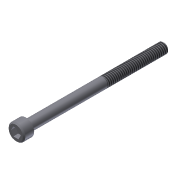
# Autodesk Inventor part: 10-32 x1000
Saved by Autodesk Inventor 2013 (Build 170138000, 138)
## iProperties
Created: 2011-07-11
Part Number: 10-32 x1000
Document SubType Name: Modeling
Designer: Dan Niemitalo
Density: 7.85 g/cm^3
Material: Steel
Mass: 5.59341 g
Surface Area: 6.83094 cm^2
Volume: 0.712536 cm^3
Author: Dan Niemitalo
Autodesk Inventor part; units mm, degrees
ref_plane "YZ Plane" through (0, 0, 0) normal (1, 0, 0) x (0, 1, 0)
ref_plane "XZ Plane" through (0, 0, 0) normal (0, 1, 0) x (-1, 0, 0)
ref_plane "XY Plane" through (0, 0, 0) normal (0, 0, 1) x (1, 0, 0)
sketch "Sketch1" plane through (0, 0, 0) normal (0, 0, 1) x (1, 0, 0)
  circle A0 centre (0, 0) radius 3.429
  dimension "d0" = 6.858
  constraints: 1 centre point, 1 coincident
  measures "d0" diameter of A0
extrude "Extrusion1" add sketch "Sketch1" along normal blind 4.1656
sketch "Sketch2" plane through (0, 0, 0) normal (0, 0, -1) x (-1, 0, 0)
  circle A0 centre (0, 0) radius 3.429 projected
  circle A1 centre (0, 0) radius 2.0828
  dimension "d3" = 4.1656
  constraints: 1 centre point, 1 coincident
  measures "d3" diameter of A1
extrude "Extrusion2" add sketch "Sketch2" along normal blind 57.15 contours A1
sketch "Sketch3" plane through (0, 0, 4.1656) normal (0, 0, 1) x (1, 0, 0)
  circle A0 centre (0, 0) radius 3.429 projected
  line L0 (-1.0311, 1.7859) -> (1.0311, 1.7859)
  line L1 (1.0311, 1.7859) -> (2.0622, 0)
  line L2 (2.0622, 0) -> (1.0311, -1.7859)
  line L3 (1.0311, -1.7859) -> (-1.0311, -1.7859)
  line L4 (-1.0311, -1.7859) -> (-2.0622, 0)
  line L5 (-2.0622, 0) -> (-1.0311, 1.7859)
  dimension "d6" = 3.5719
  constraints: 12 end point, 1 coincident, 1 horizontal, 13 other
  measures "d6" distance between parallel lines of L3 L0
extrude "Extrusion3" cut sketch "Sketch3" against normal blind 2.032 contours L0 L1 L2 L3 L4 L5
thread "Thread1" size "8-32 UNC" class "2A" standard "ANSI Unified Screw Threads" length 25.4
chamfer "Chamfer1" distance 0.508 angle 45 1 edges at (2.0828, 0, -57.15)
chamfer "Chamfer2" distance 0.508 angle 45 1 edges at (-3.429, 0, 4.1656)
body "Solid1"
